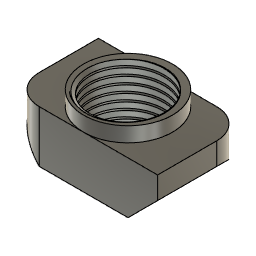
FlintZone Dock (Autodesk Fusion 360 archive; units mm, degrees)
design "M5 Nut Hammer Nut"
Autodesk Fusion 360 part; units mm, degrees
sketch "Sketch1" plane through (0, 0, 0) normal (0, 1, 0) x (1, 0, 0)
  line L0 (5, -1.75) -> (-5, -1.75)
  line L1 (-5, -1.75) -> (-5, 1.75)
  line L2 (-5, 1.75) -> (5, 1.75)
  line L3 (5, 1.75) -> (5, -1.75)
  line L4 (5, -1.75) -> (-5, 1.75) construction
  line L5 (-5, -1.75) -> (5, 1.75) construction
  dimension "d1" = 10
  dimension "d2" = 3.5
  constraint horizontal L0
  constraint perpendicular L0 L1
  constraint parallel L0 L2
  constraint parallel L1 L3
  constraint coincident L4 origin
  constraint coincident L5 origin
  measures "d1" distance of L1.end L2.end
  measures "d2" distance of L0.end L1.end
extrude "Extrude1" add sketch "Sketch1" along normal blind 6
chamfer "Chamfer1" distance 2 angle 45 2 edges at (5, 3, -1.75) (-5, 3, -1.75)
sketch "Sketch2" plane through (0, 0, 1.75) normal (0, 0, 1) x (-1, 0, 0)
  line L0 (-5, -6) -> (5, -6)
  line L1 (5, -6) -> (5, 0)
  line L2 (5, 0) -> (-5, 0)
  line L3 (-5, 0) -> (-5, -6)
  circle A0 centre (0, -3) radius 3
  constraint tangent L0 A0
extrude "Extrude2" add sketch "Sketch2" along normal blind 1 contours A0
hole "Hole1" at (0, 3, 2.75) direction (0, 0, -1) diameter 5.029 depth 18 tip angle 118
thread "Thread1" "ISO Metric profile 5.5 M5.5x0.5 6H" major diameter 5.5961 minor diameter 5.0287 pitch 0.5 angle 60 modelled right hand crest width 0.1308 on face at (0.1253, 0.4886, 1.25) crest through (2.5144, 3, 2.625)
fillet "Fillet1" radius 2 2 edges at (-5, 0, 1) (5, 6, 1)

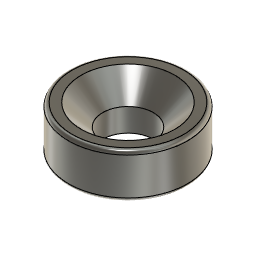
design "Magnet 8x3"
Autodesk Fusion 360 part; units mm, degrees
sketch "Sketch1" plane through (0, 0, 0) normal (0, 0, 1) x (1, 0, 0)
  circle A0 centre (0, 0) radius 4
  dimension "d1" = 8
  constraint coincident A0.centre origin
  measures "d1" diameter of A0
extrude "Extrude1" add sketch "Sketch1" along normal blind 3
hole "Hole1" at (0, 0, 3) direction (0, 0, -1) diameter 3.4 depth 8 tip angle 118 countersink diameter 6.3 countersink angle 90
fillet "Fillet1" radius 0.25 2 edges at (-3.7293, -1.4465, 0) (-3.7293, -1.4465, 3)
